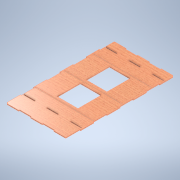
# Autodesk Inventor part: DoorFront_V2
Saved by Autodesk Inventor 2022.2 (Build 262287000, 287)
## iProperties
Created: 2022-11-15
Part Number: DoorFront_V2
Material: Generic
Document SubType Name: Modeling
Designer: jaege
Density: 1 g/cm^3
Appearance: Red Oak - Natural Low Gloss
Author: jaege
Autodesk Inventor part; units mm, degrees
ref_plane "YZ Plane" through (0, 0, 0) normal (1, 0, 0) x (0, 1, 0)
ref_plane "XZ Plane" through (0, 0, 0) normal (0, 1, 0) x (-1, 0, 0)
ref_plane "XY Plane" through (0, 0, 0) normal (0, 0, 1) x (1, 0, 0)
sketch "Sketch1" plane through (0, 0, 0) normal (0, 1, 0) x (-1, 0, 0)
  line L0 (-125, 225) -> (125, 225) construction
  line L1 (125, 225) -> (125, -225) construction
  line L2 (125, -225) -> (-125, -225) construction
  line L3 (-125, -225) -> (-125, 225) construction
  line L4 (-125, 225) -> (125, -225) construction
  line L5 (125, 225) -> (-125, -225) construction
  line L6 (125, 225) -> (75, 225) construction
  line L7 (75, 225) -> (75, 229)
  line L8 (75, 229) -> (125, 229)
  line L9 (125, 229) -> (125, 225)
  line L10 (125, 225) -> (129, 225)
  line L11 (129, 225) -> (129, 168.75)
  line L12 (129, 168.75) -> (125, 168.75)
  line L13 (125, 168.75) -> (125, 225) construction
  line L14 (-125, 225) -> (-129, 225) construction
  line L15 (-129, 225) -> (-129, 168.75) construction
  line L16 (-129, 168.75) -> (-125, 168.75)
  line L17 (-125, 168.75) -> (-125, 225)
  line L18 (125, -225) -> (75, -225) construction
  line L19 (75, -225) -> (75, -229)
  line L20 (75, -229) -> (125, -229)
  line L21 (125, -229) -> (125, -225)
  line L22 (125, 112.5) -> (125, 168.75)
  line L23 (125, 168.75) -> (129, 168.75)
  line L24 (129, 112.5) -> (125, 112.5)
  line L25 (129, 168.75) -> (129, 112.5) construction
  line L26 (-125, 112.5) -> (-125, 168.75) construction
  line L27 (-125, 168.75) -> (-129, 168.75)
  line L28 (-129, 168.75) -> (-129, 112.5)
  line L29 (-129, 112.5) -> (-125, 112.5)
  line L30 (125, 56.25) -> (125, 112.5) construction
  line L31 (125, 112.5) -> (129, 112.5)
  line L32 (129, 56.25) -> (125, 56.25)
  line L33 (129, 112.5) -> (129, 56.25)
  line L34 (-125, 56.25) -> (-125, 112.5)
  line L35 (-125, 112.5) -> (-129, 112.5)
  line L36 (-129, 112.5) -> (-129, 56.25) construction
  line L37 (-129, 56.25) -> (-125, 56.25)
  line L38 (125, 0) -> (125, 56.25)
  line L39 (125, 56.25) -> (129, 56.25)
  line L40 (129, 0) -> (125, 0)
  line L41 (129, 56.25) -> (129, 0) construction
  line L42 (-125, 0) -> (-125, 56.25) construction
  line L43 (-125, 56.25) -> (-129, 56.25)
  line L44 (-129, 56.25) -> (-129, 0)
  line L45 (-129, 0) -> (-125, 0)
  line L46 (125, -56.25) -> (125, 0) construction
  line L47 (125, 0) -> (129, 0)
  line L48 (129, -56.25) -> (125, -56.25)
  line L49 (129, 0) -> (129, -56.25)
  line L50 (-125, -56.25) -> (-125, 0)
  line L51 (-125, 0) -> (-129, 0)
  line L52 (-129, 0) -> (-129, -56.25) construction
  line L53 (-129, -56.25) -> (-125, -56.25)
  line L54 (125, -112.5) -> (125, -56.25)
  line L55 (125, -56.25) -> (129, -56.25)
  line L56 (129, -112.5) -> (125, -112.5)
  line L57 (129, -56.25) -> (129, -112.5) construction
  line L58 (-125, -112.5) -> (-125, -56.25) construction
  line L59 (-125, -56.25) -> (-129, -56.25)
  line L60 (-129, -56.25) -> (-129, -112.5)
  line L61 (-129, -112.5) -> (-125, -112.5)
  line L62 (125, -168.75) -> (125, -112.5) construction
  line L63 (125, -112.5) -> (129, -112.5)
  line L64 (129, -168.75) -> (125, -168.75)
  line L65 (129, -112.5) -> (129, -168.75)
  line L66 (-125, -168.75) -> (-125, -112.5)
  line L67 (-125, -112.5) -> (-129, -112.5)
  line L68 (-129, -112.5) -> (-129, -168.75) construction
  line L69 (-129, -168.75) -> (-125, -168.75)
  line L70 (125, -225) -> (125, -168.75)
  line L71 (125, -168.75) -> (129, -168.75)
  line L72 (129, -225) -> (125, -225) construction
  line L73 (129, -168.75) -> (129, -225) construction
  line L74 (-125, -225) -> (-125, -168.75) construction
  line L75 (-125, -168.75) -> (-129, -168.75)
  line L76 (-129, -168.75) -> (-129, -225)
  line L77 (-129, -225) -> (-125, -225)
  line L78 (75, 229) -> (75, 225)
  line L79 (25, 225) -> (25, 229)
  line L80 (25, 229) -> (75, 229) construction
  line L81 (75, 225) -> (25, 225)
  line L82 (75, -225) -> (25, -225)
  line L83 (25, -225) -> (25, -229)
  line L84 (25, -229) -> (75, -229) construction
  line L85 (75, -229) -> (75, -225)
  line L86 (25, 229) -> (25, 225)
  line L87 (-25, 225) -> (-25, 229)
  line L88 (-25, 229) -> (25, 229)
  line L89 (25, 225) -> (-25, 225) construction
  line L90 (25, -225) -> (-25, -225) construction
  line L91 (-25, -225) -> (-25, -229)
  line L92 (-25, -229) -> (25, -229)
  line L93 (25, -229) -> (25, -225)
  line L94 (-25, 229) -> (-25, 225)
  line L95 (-75, 225) -> (-75, 229)
  line L96 (-75, 229) -> (-25, 229) construction
  line L97 (-25, 225) -> (-75, 225)
  line L98 (-25, -225) -> (-75, -225)
  line L99 (-75, -225) -> (-75, -229)
  line L100 (-75, -229) -> (-25, -229) construction
  line L101 (-25, -229) -> (-25, -225)
  line L102 (-75, 229) -> (-75, 225)
  line L103 (-125, 225) -> (-125, 229)
  line L104 (-125, 229) -> (-75, 229)
  line L105 (-75, 225) -> (-125, 225) construction
  line L106 (-75, -225) -> (-125, -225) construction
  line L107 (-125, -225) -> (-125, -229)
  line L108 (-125, -229) -> (-75, -229)
  line L109 (-75, -229) -> (-75, -225)
  point P0 (0, 0)
  point P1 (75, -225)
  point P2 (25, -225)
  point P3 (-25, -225)
  point P4 (-75, -225)
  point P5 (-129, 168.75)
  point P6 (-129, 56.25)
  point P7 (-129, -168.75)
  dimension "d0" = 250
  dimension "d1" = 450
  dimension "d2" = 50
  dimension "d3" = 4
  dimension "d4" = 4
  dimension "d5" = 56.25
  dimension "d6" = 4
  dimension "d7" = 56.25
  dimension "d8" = 50
  dimension "d9" = 4
  dimension "d12" = 56.25
  dimension "d19" = 50
  constraints: 220 end point, 10 parallel, 6 horizontal, 5 perpendicular, 2 midpoint, 1 vertical, 180 other
  measures "d0" distance of L1.end L2.end
  measures "d1" distance of L0.end L1.end
  measures "d2" distance of L7.end L8.end
  measures "d3" distance of L6.end L7.end
  measures "d4" distance of L11.end L12.end
  measures "d5" distance of L10.end L11.end
  measures "d6" distance of L16.end L15.end
  measures "d7" distance of L15.end L14.end
  measures "d8" distance of L20.end L19.end
  measures "d9" distance of L19.end L18.end
  measures "d12" distance of L0.end L22.end
  measures "d19" distance of L0.end L78.end
extrude "Extrusion1" add sketch "Sketch1" along normal blind 4
sketch "Sketch2" plane through (0, 4, 0) normal (0, 1, 0) x (1, 0, 0)
  line L0 (-125, 112.5) -> (-125, 56.25) projected
  line L1 (129, 112.5) -> (125, 112.5) projected
  line L2 (-125, 112.5) -> (125, 112.5) construction
  line L3 (125, -112.5) -> (125, -56.25) projected
  line L4 (125, -56.25) -> (-125, -56.25) construction
  line L5 (-45, 127.5) -> (45, 127.5)
  line L6 (45, 127.5) -> (45, 27.5)
  line L7 (45, 27.5) -> (-45, 27.5)
  line L8 (-45, 27.5) -> (-45, 127.5)
  line L9 (-45, 127.5) -> (45, 27.5) construction
  line L10 (45, 127.5) -> (-45, 27.5) construction
  line L11 (45, -96.25) -> (-45, -96.25)
  line L12 (-45, -96.25) -> (-45, 3.75)
  line L13 (-45, 3.75) -> (45, 3.75)
  line L14 (45, 3.75) -> (45, -96.25)
  line L15 (45, -96.25) -> (-45, 3.75) construction
  line L16 (-45, -96.25) -> (45, 3.75) construction
  line L17 (25, 229) -> (-25, 229) projected
  point P0 (0, 0)
  point P1 (0, 77.5)
  point P2 (0, -46.25)
  point P3 (0, -46.25)
  point P4 (0, 77.5)
  point P5 (0, 77.5)
  point P6 (0, 229)
  point P7 (0, -46.25)
  dimension "d26" = 90
  dimension "d27" = 100
  dimension "d28" = 90
  dimension "d29" = 100
  dimension "d59" = 35
  dimension "d60" = 10
  constraints: 28 end point, 9 midpoint, 4 parallel, 3 horizontal, 2 perpendicular, 2 vertical alignment
  measures "d26" distance of L6.end L7.end
  measures "d27" distance of L5.end L6.end
  measures "d28" distance of L12.end L13.end
  measures "d29" distance of L11.end L12.end
  measures "d59" distance from line of point (0, 77.5) L2
  measures "d60" distance from line of L4 point (0, -46.25)
extrude "Extrusion2" cut sketch "Sketch2" against normal up to next
sketch "Sketch3" plane through (0, 4, 0) normal (0, 1, 0) x (1, 0, 0)
  line L0 (-129, 56.25) -> (-129, 0) projected
  line L1 (125, 0) -> (125, 56.25) projected
  line L2 (-129, 18.125) -> (125, 18.125)
  line L3 (125, 18.125) -> (125, 13.125)
  line L4 (125, 13.125) -> (-129, 13.125)
  line L5 (-129, 13.125) -> (-129, 18.125)
  line L6 (-128.3607, 15.625) -> (125.6393, 15.625) construction
  line L7 (-129, 18.125) -> (-125, 18.125)
  line L8 (-125, 18.125) -> (-125, 13.125)
  line L9 (-125, 13.125) -> (-129, 13.125)
  line L10 (-129, 13.125) -> (-129, 18.125)
  line L11 (-125, 0) -> (-125, -56.25) projected
  line L12 (45, 127.5) -> (45, 27.5) projected
  line L13 (45, 27.5) -> (-45, 27.5) projected
  line L14 (-45, 27.5) -> (-45, 127.5) projected
  line L15 (-45, 127.5) -> (45, 127.5) projected
  line L16 (-45, -96.25) -> (-45, 3.75) projected
  line L17 (-45, 3.75) -> (45, 3.75) projected
  line L18 (45, 3.75) -> (45, -96.25) projected
  line L19 (45, -96.25) -> (-45, -96.25) projected
  line L20 (-25, -225) -> (-25, -229) projected
  line L21 (-25, -229) -> (25, -229) projected
  line L22 (25, -229) -> (25, -225) projected
  line L23 (25, -225) -> (75, -225) projected
  line L24 (75, -225) -> (75, -229) projected
  line L25 (75, -229) -> (125, -229) projected
  line L26 (125, -229) -> (125, -168.75) projected
  line L27 (125, -168.75) -> (129, -168.75) projected
  line L28 (129, -168.75) -> (129, -112.5) projected
  line L29 (129, -112.5) -> (125, -112.5) projected
  line L30 (125, -112.5) -> (125, -56.25) projected
  line L31 (125, -56.25) -> (129, -56.25) projected
  line L32 (129, -56.25) -> (129, 0) projected
  line L33 (129, 0) -> (125, 0) projected
  line L34 (125, 0) -> (125, 56.25) projected
  line L35 (125, 56.25) -> (129, 56.25) projected
  line L36 (129, 56.25) -> (129, 112.5) projected
  line L37 (129, 112.5) -> (125, 112.5) projected
  line L38 (125, 112.5) -> (125, 168.75) projected
  line L39 (125, 168.75) -> (129, 168.75) projected
  line L40 (129, 168.75) -> (129, 225) projected
  line L41 (129, 225) -> (125, 225) projected
  line L42 (125, 225) -> (125, 229) projected
  line L43 (125, 229) -> (75, 229) projected
  line L44 (75, 229) -> (75, 225) projected
  line L45 (75, 225) -> (25, 225) projected
  line L46 (25, 225) -> (25, 229) projected
  line L47 (25, 229) -> (-25, 229) projected
  line L48 (-25, 229) -> (-25, 225) projected
  line L49 (-25, 225) -> (-75, 225) projected
  line L50 (-75, 225) -> (-75, 229) projected
  line L51 (-75, 229) -> (-125, 229) projected
  line L52 (-125, 229) -> (-125, 168.75) projected
  line L53 (-125, 168.75) -> (-129, 168.75) projected
  line L54 (-129, 168.75) -> (-129, 112.5) projected
  line L55 (-129, 112.5) -> (-125, 112.5) projected
  line L56 (-125, 112.5) -> (-125, 56.25) projected
  line L57 (-125, 56.25) -> (-129, 56.25) projected
  line L58 (-129, 56.25) -> (-129, 0) projected
  line L59 (-129, 0) -> (-125, 0) projected
  line L60 (-125, 0) -> (-125, -56.25) projected
  line L61 (-125, -56.25) -> (-129, -56.25) projected
  line L62 (-129, -56.25) -> (-129, -112.5) projected
  line L63 (-129, -112.5) -> (-125, -112.5) projected
  line L64 (-125, -112.5) -> (-125, -168.75) projected
  line L65 (-125, -168.75) -> (-129, -168.75) projected
  line L66 (-129, -168.75) -> (-129, -225) projected
  line L67 (-129, -225) -> (-125, -225) projected
  line L68 (-125, -225) -> (-125, -229) projected
  line L69 (-125, -229) -> (-75, -229) projected
  line L70 (-75, -229) -> (-75, -225) projected
  line L71 (-75, -225) -> (-25, -225) projected
  line L72 (-45, -96.25) -> (-45, 3.75) projected
  line L73 (-45, 27.5) -> (-45, 3.75) construction
  point P0 (0, 0)
  point P1 (125, 13.125)
  point P2 (-125, 15.625)
  point P3 (-45, 15.625)
  dimension "d32" = 5
  constraints: 20 end point, 4 parallel, 2 collinear, 2 horizontal, 2 midpoint, 2 perpendicular, 2 point on line, 1 horizontal alignment, 1 vertical, 1 other
  measures "d32" distance of L2.end L3.end
extrude "Extrusion3" cut sketch "Sketch3" against normal blind 1 contours L2 L1 L4 L8
sketch "Sketch4" plane through (0, 4, 0) normal (0, 1, 0) x (1, 0, 0)
  line L0 (-125, -110.625) -> (125, -110.625)
  line L1 (125, -110.625) -> (125, -105.625)
  line L2 (125, -105.625) -> (-125, -105.625)
  line L3 (-125, -105.625) -> (-125, -110.625)
  line L4 (-125, -110.625) -> (125, -105.625) construction
  line L5 (125, -110.625) -> (-125, -105.625) construction
  line L6 (-125, -112.5) -> (-125, -168.75) projected
  line L7 (-125, -108.125) -> (125, -108.125) construction
  line L8 (129, -168.75) -> (129, -112.5) projected
  line L9 (129, 168.75) -> (129, 225) projected
  line L10 (129, 139.375) -> (-125, 139.375) construction
  line L11 (-125, 229) -> (-125, 168.75) projected
  line L12 (-125, 136.875) -> (125, 136.875)
  line L13 (125, 136.875) -> (125, 141.875)
  line L14 (125, 141.875) -> (-125, 141.875)
  line L15 (-125, 141.875) -> (-125, 136.875)
  line L16 (-125, 136.875) -> (125, 141.875) construction
  line L17 (125, 136.875) -> (-125, 141.875) construction
  line L18 (125, 112.5) -> (125, 168.75) projected
  line L19 (-125, 229) -> (-125, 168.75) projected
  line L20 (45, 3.75) -> (-45, 3.75) projected
  line L21 (-45, 3.75) -> (-45, 13.125) construction
  line L22 (125, 13.125) -> (-125, 13.125) projected
  line L23 (-125, 13.125) -> (-125, 18.125) projected
  line L24 (-125, 18.125) -> (125, 18.125) projected
  line L25 (125, 18.125) -> (125, 56.25) projected
  line L26 (125, 56.25) -> (129, 56.25) projected
  line L27 (129, 56.25) -> (129, 112.5) projected
  line L28 (129, 112.5) -> (125, 112.5) projected
  line L29 (125, 112.5) -> (125, 168.75) projected
  line L30 (125, 168.75) -> (129, 168.75) projected
  line L31 (129, 168.75) -> (129, 225) projected
  line L32 (129, 225) -> (125, 225) projected
  line L33 (125, 225) -> (125, 229) projected
  line L34 (125, 229) -> (75, 229) projected
  line L35 (75, 229) -> (75, 225) projected
  line L36 (75, 225) -> (25, 225) projected
  line L37 (25, 225) -> (25, 229) projected
  line L38 (25, 229) -> (-25, 229) projected
  line L39 (-25, 229) -> (-25, 225) projected
  line L40 (-25, 225) -> (-75, 225) projected
  line L41 (-75, 225) -> (-75, 229) projected
  line L42 (-75, 229) -> (-125, 229) projected
  line L43 (-125, 229) -> (-125, 168.75) projected
  line L44 (-125, 168.75) -> (-129, 168.75) projected
  line L45 (-129, 168.75) -> (-129, 112.5) projected
  line L46 (-129, 112.5) -> (-125, 112.5) projected
  line L47 (-125, 112.5) -> (-125, 56.25) projected
  line L48 (-125, 56.25) -> (-129, 56.25) projected
  line L49 (-129, 56.25) -> (-129, 0) projected
  line L50 (-129, 0) -> (-125, 0) projected
  line L51 (-125, 0) -> (-125, -56.25) projected
  line L52 (-125, -56.25) -> (-129, -56.25) projected
  line L53 (-129, -56.25) -> (-129, -112.5) projected
  line L54 (-129, -112.5) -> (-125, -112.5) projected
  line L55 (-125, -112.5) -> (-125, -168.75) projected
  line L56 (-125, -168.75) -> (-129, -168.75) projected
  line L57 (-129, -168.75) -> (-129, -225) projected
  line L58 (-129, -225) -> (-125, -225) projected
  line L59 (-125, -225) -> (-125, -229) projected
  line L60 (-125, -229) -> (-75, -229) projected
  line L61 (-75, -229) -> (-75, -225) projected
  line L62 (-75, -225) -> (-25, -225) projected
  line L63 (-25, -225) -> (-25, -229) projected
  line L64 (-25, -229) -> (25, -229) projected
  line L65 (25, -229) -> (25, -225) projected
  line L66 (25, -225) -> (75, -225) projected
  line L67 (75, -225) -> (75, -229) projected
  line L68 (75, -229) -> (125, -229) projected
  line L69 (125, -229) -> (125, -168.75) projected
  line L70 (125, -168.75) -> (129, -168.75) projected
  line L71 (129, -168.75) -> (129, -112.5) projected
  line L72 (129, -112.5) -> (125, -112.5) projected
  line L73 (125, -112.5) -> (125, -56.25) projected
  line L74 (125, -56.25) -> (129, -56.25) projected
  line L75 (129, -56.25) -> (129, 0) projected
  line L76 (129, 0) -> (125, 0) projected
  line L77 (125, 0) -> (125, 13.125) projected
  line L78 (-45, -96.25) -> (-45, 3.75) projected
  line L79 (-45, 3.75) -> (45, 3.75) projected
  line L80 (45, 3.75) -> (45, -96.25) projected
  line L81 (45, -96.25) -> (-45, -96.25) projected
  line L82 (45, 127.5) -> (45, 27.5) projected
  line L83 (45, 27.5) -> (-45, 27.5) projected
  line L84 (-45, 27.5) -> (-45, 127.5) projected
  line L85 (-45, 127.5) -> (45, 127.5) projected
  line L86 (-45, -96.25) -> (-45, 3.75) projected
  line L87 (-45, -96.25) -> (-45, -105.625) construction
  line L88 (125, 13.125) -> (-125, 13.125) projected
  line L89 (-45, 127.5) -> (-45, 27.5) projected
  line L90 (-45, 127.5) -> (-45, 136.875) construction
  point P0 (0, 0)
  point P1 (0, -108.125)
  point P2 (0, 139.375)
  point P3 (-125, 183.1313)
  point P4 (-125, 178.1313)
  dimension "d36" = 5
  dimension "d39" = 5
  constraints: 34 end point, 7 midpoint, 5 perpendicular, 5 point on line, 4 collinear, 4 parallel, 3 horizontal, 3 vertical alignment, 1 vertical
  measures "d36" distance of L0.end L1.end
  measures "d39" distance of L12.end L13.end
extrude "Extrusion4" cut sketch "Sketch4" against normal blind 1 contours L3 L2 L1 L0 | L12 L15 L14 L13
sketch "Sketch5" plane through (0, 4, 0) normal (0, 1, 0) x (1, 0, 0)
  line L0 (-125, -158) -> (-75, -158)
  line L1 (-75, -158) -> (-75, -162)
  line L2 (-75, -162) -> (-125, -162)
  line L3 (-125, -162) -> (-125, -158)
  line L4 (-75, -225) -> (-25, -225) projected
  line L5 (-125, -112.5) -> (-125, -168.75) projected
  line L6 (125, -110.625) -> (-125, -110.625) projected
  line L7 (-75, -158) -> (-25, -158)
  line L8 (-25, -158) -> (-25, -162)
  line L9 (-25, -162) -> (-75, -162)
  line L10 (-75, -162) -> (-75, -158)
  line L11 (-25, -158) -> (25, -158)
  line L12 (25, -158) -> (25, -162)
  line L13 (25, -162) -> (-25, -162)
  line L14 (-25, -162) -> (-25, -158)
  line L15 (25, -158) -> (75, -158)
  line L16 (75, -158) -> (75, -162)
  line L17 (75, -162) -> (25, -162)
  line L18 (25, -162) -> (25, -158)
  line L19 (75, -158) -> (125, -158)
  line L20 (125, -158) -> (125, -162)
  line L21 (125, -162) -> (75, -162)
  line L22 (75, -162) -> (75, -158)
  line L23 (-25, 188) -> (-75, 188)
  line L24 (-75, 192) -> (-25, 192)
  line L25 (-25, 192) -> (-25, 188)
  line L26 (-25, 188) -> (-25, 192)
  line L27 (25, 188) -> (-25, 188)
  line L28 (-25, 192) -> (25, 192)
  line L29 (25, 192) -> (25, 188)
  line L30 (25, 188) -> (25, 192)
  line L31 (25, 192) -> (75, 192)
  line L32 (75, 188) -> (25, 188)
  line L33 (-75, 192) -> (-75, 188)
  line L34 (-75, 188) -> (-75, 192)
  line L35 (-125, 192) -> (-75, 192)
  line L36 (-125, 188) -> (-125, 192)
  line L37 (-75, 188) -> (-125, 188)
  line L38 (75, 192) -> (75, 188)
  line L39 (75, 188) -> (75, 192)
  line L40 (75, 192) -> (125, 192)
  line L41 (125, 192) -> (125, 188)
  line L42 (125, 188) -> (75, 188)
  point P0 (0, 0)
  point P1 (125, -143.125)
  point P2 (-125, -110.625)
  dimension "d40" = 50
  dimension "d41" = 4
  dimension "d42" = 63
  dimension "d45" = 50
  dimension "d54" = 350
  constraints: 80 end point, 16 horizontal alignment, 10 parallel, 8 collinear, 1 horizontal, 1 perpendicular, 1 vertical, 41 other
  measures "d40" distance of L1.end L2.end
  measures "d41" distance of L0.end L1.end
  measures "d42" distance between parallel lines of L4 L2
  measures "d45" distance of L0.start L7.start
  measures "d54" distance of L8.end L23.start
extrude "Extrusion5" cut sketch "Sketch5" against normal up to next contours L0 L1 L2 L3 | L11 L12 L13 L8 | L19 L20 L21 L16 | L25 L28 L29 L27 | L37 L36 L35 L33 | L38 L40 L41 L42
body "Solid1"
